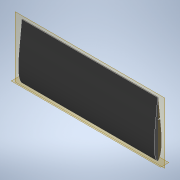
# Autodesk Inventor part: IISRD_Wing_Control_surface
Saved by Autodesk Inventor 2021 (Build 250183000, 183)
## iProperties
Created: 2020-10-19
Part Number: IISRD_Wing_Control_surface
Material: EPP Foam
Document SubType Name: Modeling
Designer: Kanenas
Mass: 7.60891 g
Surface Area: 754.445 cm^2
Volume: 380.446 cm^3
Density: 0.02 g/cm^3
Appearance: Generic
Author: Kanenas
Autodesk Inventor part; units mm, degrees
ref_plane "YZ Plane" through (0, 0, 0) normal (1, 0, 0) x (0, 1, 0)
sketch "Sketch1" plane through (0, 0, 0) normal (1, 0, 0) x (0, 1, 0)
  spline S0 degree 5 poles (140, 0) (140, 0.008) (139.6909, 0.023) (138.2456, 0.0648) (138.0851, 0.2448) (134.3445, 0.4509) (132.587, 0.7525) (128.0169, 1.03) (124.0758, 1.4239) (118.6617, 1.8648) (113.1342, 2.4056) (106.871, 3.0117) (100.3305, 3.6855) (93.4209, 4.4087) (86.3255, 5.1563) (79.0958, 5.9053) (71.8372, 6.629) (64.6288, 7.2884) (57.549, 7.8613) (50.671, 8.3132) (44.0585, 8.6184) (37.7676, 8.751) (31.8409, 8.7076) (26.336, 8.4735) (21.2773, 8.0467) (16.7064, 7.4272) (12.6313, 6.6359) (9.1041, 5.7147) (6.0909, 4.6974) (3.705, 3.6163) (1.758, 2.4782) (0.495, 1.2916) (-0.4137, 0) (0.495, -1.2916) (1.758, -2.4782) (3.705, -3.6163) (6.0909, -4.6974) (9.1041, -5.7147) (12.6313, -6.6359) (16.7064, -7.4272) (21.2773, -8.0467) (26.336, -8.4735) (31.8409, -8.7076) (37.7676, -8.751) (44.0585, -8.6184) (50.671, -8.3132) (57.549, -7.8613) (64.6288, -7.2884) (71.8372, -6.629) (79.0958, -5.9053) (86.3255, -5.1563) (93.4209, -4.4087) (100.3305, -3.6855) (106.871, -3.0117) (113.1342, -2.4056) (118.6617, -1.8648) (124.0758, -1.4239) (128.0169, -1.03) (132.587, -0.7525) (134.3445, -0.4509) (138.0851, -0.2448) (138.2456, -0.0648) (139.6909, -0.023) (140, -0.008) (140, 0) knots 0 0 0 0 0 0 0.009495 0.017637 0.028865 0.042353 0.057559 0.074188 0.092027 0.110874 0.13054 0.150849 0.171639 0.192755 0.214053 0.235397 0.256657 0.277714 0.298457 0.318784 0.338597 0.357809 0.37634 0.394116 0.411062 0.427101 0.442142 0.456085 0.468809 0.480163 0.490364 0.5 0.509636 0.519837 0.531191 0.543915 0.557858 0.572899 0.588938 0.605884 0.62366 0.642191 0.661403 0.681216 0.701543 0.722286 0.743343 0.764603 0.785947 0.807245 0.828361 0.849151 0.86946 0.889126 0.907973 0.925812 0.942441 0.957647 0.971135 0.982363 0.990505 1 1 1 1 1 1
  line L0 (130, 16.3724) -> (164.1986, 16.3724)
  line L1 (164.1986, 16.3724) -> (164.1986, -9.4783)
  line L2 (164.1986, -9.4783) -> (130, -9.4783)
  line L3 (130, -9.4783) -> (130, 16.3724)
  point P0 (138.0834, 0.1512)
  point P1 (135.8252, 0.3794)
  point P2 (132.797, 0.6664)
  point P3 (129.0044, 0.9884)
  point P4 (124.4796, 1.3706)
  point P5 (119.294, 1.8284)
  point P6 (113.526, 2.3674)
  point P7 (107.2624, 2.982)
  point P8 (100.5956, 3.661)
  point P9 (93.6194, 4.389)
  point P10 (86.4304, 5.1422)
  point P11 (79.1224, 5.8954)
  point P12 (71.785, 6.6192)
  point P13 (64.505, 7.28)
  point P14 (57.3608, 7.8484)
  point P15 (50.4266, 8.2936)
  point P16 (43.7668, 8.5876)
  point P17 (37.4346, 8.7094)
  point P18 (31.479, 8.6478)
  point P19 (25.9504, 8.393)
  point P20 (20.881, 7.9408)
  point P21 (16.2974, 7.2954)
  point P22 (12.222, 6.4778)
  point P23 (8.6772, 5.5216)
  point P24 (5.6966, 4.4618)
  point P25 (3.3082, 3.332)
  point P26 (1.533, 2.17)
  point P27 (0.4018, 1.0262)
  point P28 (0, 0)
  point P29 (0.4018, -1.0262)
  point P30 (1.533, -2.17)
  point P31 (3.3082, -3.332)
  point P32 (5.6966, -4.4618)
  point P33 (8.6772, -5.5216)
  point P34 (12.222, -6.4778)
  point P35 (16.2974, -7.2954)
  point P36 (20.881, -7.9408)
  point P37 (25.9504, -8.393)
  point P38 (31.479, -8.6478)
  point P39 (37.4346, -8.7094)
  point P40 (43.7668, -8.5876)
  point P41 (50.4266, -8.2936)
  point P42 (57.3608, -7.8484)
  point P43 (64.505, -7.28)
  point P44 (71.785, -6.6192)
  point P45 (79.1224, -5.8954)
  point P46 (86.4304, -5.1422)
  point P47 (93.6194, -4.389)
  point P48 (100.5956, -3.661)
  point P49 (107.2624, -2.982)
  point P50 (113.526, -2.3674)
  point P51 (119.294, -1.8284)
  point P52 (124.4796, -1.3706)
  point P53 (129.0044, -0.9884)
  point P54 (132.797, -0.6664)
  point P55 (135.8252, -0.3794)
  point P56 (138.0834, -0.1512)
  point P57 (139.5086, -0.0294)
  point P58 (130, -0.9104)
  point P59 (130, 0.9104)
  dimension "d9" = 130
  constraints: 8 end point, 2 parallel, 1 horizontal, 1 perpendicular, 120 other
  measures "d9" distance from line of L3 point (0, 0)
extrude "Extrusion1" add sketch "Sketch1" along normal blind 320 contours L3 S0 picked at (63.1596, 2.072)
sketch "Sketch3" plane through (0, 0, 0) normal (0, 0, 1) x (1, 0, 0)
  line L0 (0, 130) -> (320, 130) projected
  line L1 (0, 130) -> (0, 0)
  line L2 (260, 67.75) -> (260, 62.25) projected
  line L3 (104, 130) -> (260, 130)
  line L4 (260, 130) -> (260, 91)
  line L5 (260, 91) -> (104, 91)
  line L6 (104, 91) -> (104, 130)
  dimension "d11" = 260
  dimension "d12" = 130
  dimension "d13" = 39
  dimension "d14" = 156
  constraints: 10 end point, 2 parallel, 1 horizontal, 1 perpendicular, 1 point on line
  measures "d11" distance between parallel lines of L1 L2
  measures "d12" distance of L0.start L1.end
  measures "d13" distance of L5.end L3.start
  measures "d14" distance of L4.end L5.end
sketch "Sketch4" plane through (320, 0, 0) normal (1, 0, 0) x (0, 0, -1)
  line L0 (-5.3951, 84) -> (5.3822, 84)
  line L1 (-1.3951, 84) -> (11.6611, 87.4984)
  line L2 (-1.3951, 84) -> (11.0685, 80.6604)
  line L3 (9.6415, 86.9572) -> (10.196, 80.8942)
  line L4 (7.0359, 23.8522) -> (9.6415, 23.8522)
  line L5 (9.6415, 23.8522) -> (9.6415, 28.1915)
  line L6 (9.6415, 28.1915) -> (7.0359, 28.1915)
  line L7 (7.0359, 28.1915) -> (7.0359, 23.8522)
  point P0 (0, 0)
  dimension "d17" = 84
  dimension "d18" = 4
  dimension "d19" = 15
  dimension "d20" = 15
  constraints: 16 end point, 2 horizontal, 2 parallel, 2 point on line, 1 perpendicular, 1 other
  measures "d17" vertical distance of point (0, 0) L1.start
  measures "d18" distance of L1.start L0.start
  measures "d19" angle of L1 L0
  measures "d20" angle of L0 L2
extrude "Extrusion3" cut sketch "Sketch4" against normal through all contours L1 L3 L2
ref_plane "Work Plane3" through (160, 36.3757, 8.7122) normal (0, 0, 1) x (1, 0, 0)
fillet "Fillet1" radius 0.5 1 edges at (160, 84, 1.3951)
ref_plane "Work Plane4" through (160, 36.3757, -8.7122) normal (0, 0, -1) x (-1, 0, 0)
sketch "Sketch13" plane through (160, 36.3757, -8.7122) normal (0, 0, -1) x (-1, 0, 0)
  line L0 (-48.6, 25.6243) -> (-40, 25.6243)
  line L1 (-40, 25.6243) -> (-40, -2.3757)
  line L2 (-40, -2.3757) -> (-48.6, -2.3757)
  line L3 (-48.6, -2.3757) -> (-48.6, 25.6243)
  point P0 (160, -36.3757)
  dimension "d67" = 200
  dimension "d68" = 8.6
  dimension "d69" = 28
  dimension "d70" = 34
  constraints: 8 end point, 2 parallel, 1 horizontal, 1 perpendicular
  measures "d67" distance from line of L1 point (160, -36.376)
  measures "d68" distance of L0.start L0.end
  measures "d69" distance of L2.end L0.start
  measures "d70" distance from line of L2 point (160, -36.376)
extrude "Extrusion9" cut sketch "Sketch13" against normal blind 2
sketch "Sketch14" plane through (160, 36.3757, -8.7122) normal (0, 0, -1) x (-1, 0, 0)
  line L0 (-61, 66.4157) -> (-60, 66.4157)
  line L1 (-60, 66.4157) -> (-60, 86.4157)
  line L2 (-60, 86.4157) -> (-61, 86.4157)
  line L3 (-61, 86.4157) -> (-61, 66.4157)
  point P0 (160, -36.3757)
  dimension "d73" = 220
  dimension "d74" = 1
  dimension "d75" = 20
  constraints: 8 end point, 2 parallel, 1 horizontal, 1 perpendicular
  measures "d73" distance from line of L1 point (160, -36.376)
  measures "d74" distance of L1.end L2.end
  measures "d75" distance of L2.end L0.start
extrude "Extrusion10" cut sketch "Sketch14" against normal blind 8
equation "\"d13\" = 0.3 * d12"
equation "\"d14\" = 0.6 * d11"
body "Solid1"
